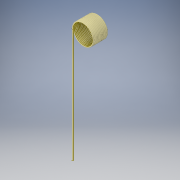
# Autodesk Inventor part: Winding
Saved by Autodesk Inventor 2016 (Build 200138000, 138)
## iProperties
Created: 2016-04-11
Part Number: Winding
Material: Nylon 6/6
Document SubType Name: Modeling
Designer: agmle
Density: 1.13 g/cm^3
Appearance: Nylon 6
Author: agmle
Autodesk Inventor part; units mm, degrees
ref_plane "YZ Plane" through (0, 0, 0) normal (1, 0, 0) x (0, 1, 0)
ref_plane "XZ Plane" through (0, 0, 0) normal (0, 1, 0) x (-1, 0, 0)
ref_plane "XY Plane" through (0, 0, 0) normal (0, 0, 1) x (1, 0, 0)
sketch "Sketch1" plane through (0, 0, 0) normal (0, 1, 0) x (-1, 0, 0)
  arc A0 (-1.4605, -0.6222) -> (-1.4605, 0.6222) centre (0, 0) ccw
  line L0 (-26.8605, 0) -> (-26.8605, -65.0164) construction
  line L1 (-1.4605, 0.6222) -> (-1.4605, -0.6222)
  dimension "d0" = 3.175
  dimension "d10" = 3.048
  dimension "d11" = 25.4
  constraints: 4 end point, 2 point on circle, 2 vertical, 1 centre point, 1 coincident
  measures "d0" diameter of A0
  measures "d11" distance between parallel lines of L0 L1
coil "Coil1" sketch "Sketch1" operation add axis through (26.8605, 0, 0) along (0, 0, -1) pitch 3.302 turns 11.75 hand right
sketch "Sketch3" plane through (0, 0, 0) normal (0, -1, 0) x (1, 0, 0)
  arc A0 (1.4605, 0.6222) -> (1.4605, -0.6222) centre (0, 0) ccw projected
  line L0 (1.4605, -0.6222) -> (1.4605, 0.6222) projected
  point P0 (0, 0)
extrude "Extrusion1" add sketch "Sketch3" along normal blind 304.8
body "Solid1"
